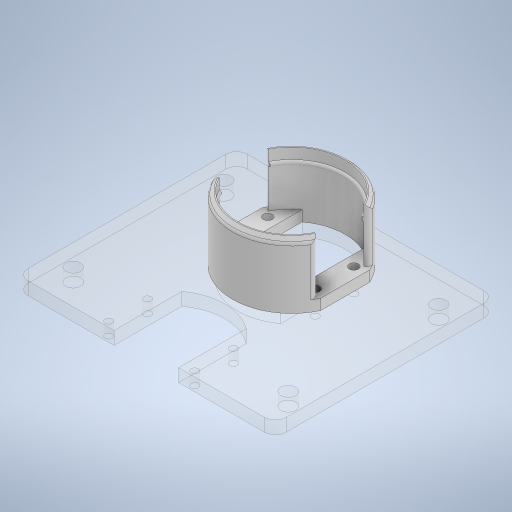
# Autodesk Inventor part: Module-EstimFloSingle
Saved by Autodesk Inventor 2023 (Build 270158000, 158)
## iProperties
Created: 2024-07-10
Part Number: Module-EstimFloSingle
Material: Generic
Document SubType Name: Modeling
Designer: incep
Density: 1 g/cm^3
Appearance: Default
Author: incep
## iProperties of the stored document Module-EstimFloSinlge_3DPrint.ipt
Created: 2024-07-10
Part Number: Module-EstimFloSinlge_3DPrint
Material: Generic
Document SubType Name: Modeling
Designer: incep
Density: 1 g/cm^3
Appearance: Default
Author: incep
Autodesk Inventor part; units mm, degrees
ref_plane "YZ Plane" through (0, 0, 0) normal (1, 0, 0) x (0, 1, 0)
ref_plane "XZ Plane" through (0, 0, 0) normal (0, 1, 0) x (-1, 0, 0)
ref_plane "XY Plane" through (0, 0, 0) normal (0, 0, 1) x (1, 0, 0)
sketch "Sketch1" plane through (0, 0, 0) normal (0, 1, 0) x (-1, 0, 0)
  line L0 (0, -75.5) -> (0, 75.5) construction
  line L1 (26.5, -75.5) -> (26.5, 75.5) construction
  line L2 (-26.5, 75.5) -> (-26.5, -75.5) construction
  arc A0 (-26.5, -75.5) -> (26.5, -75.5) centre (0, -75.5) ccw construction
  arc A1 (26.5, 75.5) -> (-26.5, 75.5) centre (0, 75.5) ccw construction
  line L3 (25, -99.5) -> (-25, -99.5)
  line L4 (-25, -99.5) -> (-25, -44.5)
  line L5 (-25, -44.5) -> (25, -44.5)
  line L6 (25, -44.5) -> (25, -99.5)
  point P0 (0, 0)
  point P1 (0, 0)
  point P2 (0, -99.5)
  dimension "d0" = 151
  dimension "d1" = 26.5
  dimension "d5" = 50
  dimension "d6" = 55
  dimension "d49" = 24
  constraints: 16 end point, 4 point on circle, 4 tangent, 3 parallel, 2 centre point, 2 midpoint, 1 coincident, 1 horizontal, 1 perpendicular, 1 vertical, 1 vertical alignment
  measures "d0" distance of L0.start L0.end
  measures "d1" radius of A0
  measures "d5" distance of L3.start L3.end
  measures "d6" distance of L5.end L3.start
  measures "d49" distance from line of L3 L0.start
extrude "Extrusion1" add sketch "Sketch1" along normal blind 5
sketch "Sketch2" plane through (0, 5, 0) normal (0, 1, 0) x (1, 0, 0)
  circle A0 centre (0, 72) radius 24.95
  line L0 (-25, 44.5) -> (25, 44.5) projected
  line L1 (25, 44.5) -> (25, 99.5) projected
  line L2 (25, 99.5) -> (-25, 99.5) projected
  line L3 (-25, 99.5) -> (-25, 44.5) projected
  circle A1 centre (0, 72) radius 27.45
  point P0 (0, 0)
  point P1 (0, 44.5)
  point P2 (25, 72)
  dimension "d9" = 49.9
  dimension "d10" = 2.5
  constraints: 2 centre point, 2 midpoint, 1 horizontal alignment, 1 vertical alignment
  measures "d9" diameter of A0
  measures "d10" radial gap between concentric circles of A0 A1
extrude "Extrusion2" add sketch "Sketch2" along normal blind 25 contours A1 L3 | L3 A1 L1 | L1 A1
sketch "Sketch3" plane through (0, 0, 0) normal (1, 0, 0) x (0, 1, 0)
  line L0 (30, -47.05) -> (30, -96.95) projected
  line L1 (5, -96.95) -> (5, -47.05) projected
  line L2 (30, -47.05) -> (30, -96.95) construction
  line L3 (30, -47.05) -> (5, -47.05) construction
  line L4 (30, -47.05) -> (5, -47.05) construction
  circle A0 centre (24, -47.05) radius 1
  line L5 (5, -72) -> (30, -72) construction
  point P0 (0, 0)
  dimension "d13" = 2
  dimension "d14" = 6
  constraints: 4 end point, 2 midpoint, 1 centre point, 1 perpendicular, 1 point on line
  measures "d13" diameter of A0
  measures "d14" distance from line of L2 A0.centre
revolve "Revolution1" add sketch "Sketch3" angle 360 about axis through (0, 5, -72) along (0, 1, 0)
sketch "Sketch4" plane through (0, 5, -72) normal (0, 1, 0) x (1, 0, 0)
  line L0 (-35, -11.3359) -> (35, -11.3359)
  line L1 (35, -11.3359) -> (35, 11.3359)
  line L2 (35, 11.3359) -> (-35, 11.3359)
  line L3 (-35, 11.3359) -> (-35, -11.3359)
  line L4 (25, 27.5) -> (-25, 27.5) construction
  line L5 (-25, 27.5) -> (-25, 11.3359) construction
  line L6 (-25, -11.3359) -> (-25, -27.5) construction
  line L7 (-25, -27.5) -> (25, -27.5) construction
  line L8 (25, -27.5) -> (25, -11.3359) construction
  line L9 (25, 11.3359) -> (25, 27.5) construction
  line L10 (-25, 11.3359) -> (-25, -11.3359) construction
  line L11 (25, -11.3359) -> (25, 11.3359) construction
  point P0 (0, -72)
  point P1 (0, 11.3359)
  point P2 (0, 27.5)
  point P3 (35, 0)
  point P4 (25, 0)
  dimension "d16" = 70
  constraints: 8 end point, 4 midpoint, 2 horizontal alignment, 2 parallel, 1 horizontal, 1 perpendicular, 1 vertical alignment
  measures "d16" distance of L1.end L2.end
extrude "Extrusion3" cut sketch "Sketch4" along normal up to surface (25 mm away)
sketch "Sketch5" plane through (0, 5, 0) normal (0, 1, 0) x (1, 0, 0)
  arc A0 (22.2261, 83.3359) -> (-22.2261, 83.3359) centre (0, 72) ccw projected
  circle A1 centre (0, 72) radius 24.95
  line L0 (-15, 99.5) -> (15, 99.5)
  line L1 (15, 99.5) -> (15, 44.5)
  line L2 (15, 44.5) -> (-15, 44.5)
  line L3 (-15, 44.5) -> (-15, 99.5)
  line L4 (25, 99.5) -> (-25, 99.5) projected
  point P0 (0, 0)
  point P1 (0, 99.5)
  point P2 (15, 72)
  point P3 (-15, 91.9375)
  point P4 (-15, 52.0625)
  point P5 (15, 52.0625)
  point P6 (15, 91.9375)
  dimension "d20" = 30
  constraints: 8 end point, 2 midpoint, 2 parallel, 1 centre point, 1 coincident, 1 collinear, 1 concentric, 1 horizontal, 1 horizontal alignment, 1 perpendicular, 1 vertical alignment
  measures "d20" distance of L0.start L0.end
extrude "Extrusion4" cut sketch "Sketch5" against normal up to surface (5 mm away) contours L1 A1 L3 A0
chamfer "Chamfer1" distance 2 angle 45 2 edges at (0, 30, -99.45) (0, 30, -44.55)
fillet "Fillet1" radius 2 6 edges at (0, 28, -44.55) (0, 28, -99.45) (-25, 16.5, -83.3359) (-25, 16.5, -60.6641) (25, 16.5, -60.6641) (25, 16.5, -83.3359)
sketch "Sketch6" plane through (0, 5, 0) normal (0, 1, 0) x (1, 0, 0)
  line L0 (25, 44.5) -> (25, 99.5) projected
  line L1 (25, 99.5) -> (-25, 99.5) projected
  line L2 (-25, 99.5) -> (-25, 44.5) projected
  line L3 (-25, 44.5) -> (25, 44.5) projected
  arc A0 (22.1915, 83.4034) -> (23.3796, 86.3839) centre (21.6762, 85.3359) ccw projected
  arc A1 (22.1915, 83.4034) -> (15, 91.9375) centre (0, 72) ccw projected
  line L4 (15, 91.9375) -> (15, 52.0625) projected
  arc A2 (15, 52.0625) -> (22.1915, 60.5966) centre (0, 72) ccw projected
  arc A3 (23.3796, 57.6161) -> (22.1915, 60.5966) centre (21.6762, 58.6641) ccw projected
  arc A4 (-23.3796, 57.6161) -> (23.3796, 57.6161) centre (0, 72) ccw projected
  arc A5 (-22.1915, 60.5966) -> (-23.3796, 57.6161) centre (-21.6762, 58.6641) ccw projected
  arc A6 (-22.1915, 60.5966) -> (-15, 52.0625) centre (0, 72) ccw projected
  line L5 (-15, 52.0625) -> (-15, 91.9375) projected
  arc A7 (-15, 91.9375) -> (-22.1915, 83.4034) centre (0, 72) ccw projected
  arc A8 (-23.3796, 86.3839) -> (-22.1915, 83.4034) centre (-21.6762, 85.3359) ccw projected
  arc A9 (23.3796, 86.3839) -> (-23.3796, 86.3839) centre (0, 72) ccw projected
  circle A10 centre (-20, 63) radius 2.1
  circle A11 centre (-20, 63) radius 3.5 construction
  line L6 (-20, 63) -> (20, 63) construction
  line L7 (20, 63) -> (20, 81) construction
  line L8 (20, 81) -> (-20, 81) construction
  line L9 (-20, 81) -> (-20, 63) construction
  circle A12 centre (20, 63) radius 2.1
  circle A13 centre (20, 81) radius 2.1
  circle A14 centre (-20, 81) radius 2.1
  point P0 (0, 0)
  point P1 (0, 63)
  point P2 (20, 72)
  dimension "d28" = 4.2
  dimension "d29" = 7
  dimension "d38" = 40
  dimension "d39" = 18
  constraints: 8 end point, 5 centre point, 4 coincident, 3 equal radius, 2 midpoint, 2 parallel, 1 horizontal, 1 horizontal alignment, 1 perpendicular, 1 vertical alignment
  measures "d28" diameter of A10
  measures "d29" diameter of A11
  measures "d38" distance of L6.start L6.end
  measures "d39" distance of L6.end L7.end
extrude "Extrusion5" cut sketch "Sketch6" against normal up to surface (5 mm away) contours A10 | A12 | A13 | A14
sketch "Sketch8" plane through (0, 5, 0) normal (0, 1, 0) x (1, 0, 0)
  arc A0 (23.3796, 86.3839) -> (-23.3796, 86.3839) centre (0, 72) ccw projected
  circle A1 centre (0, 72) radius 27.45
  arc A2 (22.1915, 83.4034) -> (15, 91.9375) centre (0, 72) ccw projected
  circle A3 centre (0, 72) radius 42.45
  point P0 (0, 0)
  dimension "d40" = 15
  constraints: 2 centre point, 1 coincident, 1 concentric
  measures "d40" radial gap between concentric circles of A1 A3
extrude "Extrusion6" cut sketch "Sketch8" against normal up to surface (5 mm away)
sketch "Sketch7" plane through (0, 0, 0) normal (0, 1, 0) x (-1, 0, 0)
  line L0 (60, -106.5) -> (-60, -106.5)
  line L1 (-60, -106.5) -> (-60, -4.5)
  line L2 (-60, -4.5) -> (60, -4.5)
  line L3 (60, -4.5) -> (60, -106.5)
  line L4 (50, -90.5) -> (-50, -90.5) construction
  line L5 (-50, -90.5) -> (-50, -20.5) construction
  line L6 (-50, -20.5) -> (50, -20.5) construction
  line L7 (50, -20.5) -> (50, -90.5) construction
  circle A0 centre (50, -20.5) radius 3.4
  circle A1 centre (50, -90.5) radius 3.4
  circle A2 centre (-50, -90.5) radius 3.4
  circle A3 centre (-50, -20.5) radius 3.4
  arc A4 (-26.5, -75.5) -> (26.5, -75.5) centre (0, -75.5) ccw construction
  point P0 (0, 0)
  point P1 (0, -106.5)
  point P2 (0, -90.5)
  point P3 (-50, -55.5)
  point P4 (-60, -55.5)
  dimension "d33" = 102
  dimension "d34" = 120
  dimension "d44" = 100
  dimension "d45" = 70
  dimension "d46" = 6.8
  dimension "d47" = 20
  constraints: 16 end point, 4 centre point, 4 coincident, 4 midpoint, 4 parallel, 3 equal radius, 2 horizontal, 2 perpendicular, 2 vertical alignment, 1 horizontal alignment
  measures "d33" distance of L0.end L1.end
  measures "d34" distance of L1.end L2.end
  measures "d44" distance of L5.end L6.end
  measures "d45" distance of L4.end L5.end
  measures "d46" diameter of A0
  measures "d47" vertical distance of point (-60, -55.5) A4.centre
extrude "Extrusion7" add sketch "Sketch7" against normal blind 6 separate body
sketch "Sketch9" plane through (0, 0, 0) normal (0, 1, 0) x (1, 0, 0)
  arc A0 (15, 91.9375) -> (-15, 91.9375) centre (0, 72) ccw projected
  line L0 (-15, 91.9375) -> (-15, 52.0625) projected
  line L1 (15, 52.0625) -> (15, 91.9375) projected
  arc A1 (-15, 52.0625) -> (15, 52.0625) centre (0, 72) ccw projected
  point P0 (0, 0)
extrude "Extrusion8" cut sketch "Sketch9" against normal up to surface (6 mm away) bodies 2
sketch "Sketch10" plane through (0, 0, 0) normal (0, 1, 0) x (1, 0, 0)
  circle A0 centre (-20, 81) radius 2.1 projected
  circle A1 centre (-20, 81) radius 1.7
  circle A2 centre (20, 81) radius 2.1 projected
  circle A3 centre (20, 81) radius 1.7
  circle A4 centre (-20, 63) radius 2.1 projected
  circle A5 centre (-20, 63) radius 1.7
  circle A6 centre (20, 63) radius 2.1 projected
  circle A7 centre (20, 63) radius 1.7
  point P0 (0, 0)
  dimension "d54" = 3.4
  constraints: 4 centre point, 4 coincident, 3 equal radius
  measures "d54" diameter of A1
extrude "Extrusion9" cut sketch "Sketch10" against normal up to surface (6 mm away) contours A1 | A3 | A5 | A7 bodies 2
pattern_linear "Rectangular Pattern1" count 2 spacing 56 along (0, 0, 1) of "Extrusion8", "Extrusion9" bodies 2
fillet "Fillet3" radius 5 4 edges at (-60, -3, -4.5) (60, -3, -4.5) (-60, -3, -106.5) (60, -3, -106.5)
